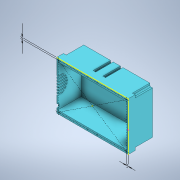
# Autodesk Inventor part: caseUpperPortion
Saved by Autodesk Inventor 2022.1 (Build 261234020, 234B)
## iProperties
Created: 2021-08-20
Part Number: caseUpperPortion
Material: PC/ABS Plastic
Document SubType Name: Modeling
Designer: robst
Density: 0.357273 g/cm^3
Appearance: Cadet Blue
Author: robst
Autodesk Inventor part; units mm, degrees
ref_plane "YZ Plane" through (0, 0, 0) normal (1, 0, 0) x (0, 1, 0)
ref_plane "XZ Plane" through (0, 0, 0) normal (0, 1, 0) x (-1, 0, 0)
ref_plane "XY Plane" through (0, 0, 0) normal (0, 0, 1) x (1, 0, 0)
sketch "Sketch1" plane through (0, 0, 0) normal (0, 0, 1) x (1, 0, 0)
  line L0 (-110.35, -74.5) -> (110.35, -74.5)
  line L1 (110.35, -74.5) -> (110.35, 74.5)
  line L2 (110.35, 74.5) -> (-110.35, 74.5)
  line L3 (-110.35, 74.5) -> (-110.35, -74.5)
  line L4 (-110.35, -74.5) -> (110.35, 74.5) construction
  line L5 (110.35, -74.5) -> (-110.35, 74.5) construction
  point P0 (0, 0)
  dimension "d0" = 220.7
  dimension "d1" = 149
  constraints: 12 end point, 2 midpoint, 2 parallel, 1 horizontal, 1 perpendicular
  measures "d0" distance of L0.start L0.end
  measures "d1" distance of L1.end L0.end
extrude "MainInnerBodyExtrusion" add sketch "Sketch1" against normal blind 75
sketch "Sketch3" plane through (0, 0, 0) normal (0, 0, 1) x (1, 0, 0)
  line L0 (37.65, -26) -> (94.65, -26)
  line L1 (94.65, -26) -> (94.65, 26)
  line L2 (94.65, 26) -> (37.65, 26)
  line L3 (37.65, 26) -> (37.65, -26)
  line L4 (37.65, -26) -> (94.65, 26) construction
  line L5 (94.65, -26) -> (37.65, 26) construction
  line L6 (110.35, -74.5) -> (110.35, 74.5) projected
  line L7 (0, 0) -> (110.35, 0) construction
  line L8 (-110.35, -74.5) -> (-110.35, 74.5) construction
  line L9 (-110.35, 74.5) -> (-110.35, -74.5) projected
  point P0 (66.15, 0)
  point P1 (66.15, 0)
  dimension "d5" = 15.7
  dimension "d6" = 52
  dimension "d7" = 57
  constraints: 14 end point, 4 midpoint, 2 parallel, 1 horizontal, 1 perpendicular, 1 point on line
  measures "d5" distance between parallel lines of L1 L6
  measures "d6" distance of L0.end L1.end
  measures "d7" distance of L1.end L2.end
extrude "HoleForCamerabase" cut sketch "Sketch3" against normal blind 47
sketch "Sketch4" plane through (0, 0, 0) normal (0, 0, 1) x (1, 0, 0)
  line L0 (0, 0) -> (-110.35, 0) construction
  line L1 (-110.35, -74.5) -> (-110.35, 74.5) construction
  line L2 (-107.35, -31) -> (-91.35, -31)
  line L3 (-91.35, -31) -> (-91.35, 31)
  line L4 (-91.35, 31) -> (-107.35, 31)
  line L5 (-107.35, 31) -> (-107.35, -31)
  line L6 (-107.35, -31) -> (-91.35, 31) construction
  line L7 (-91.35, -31) -> (-107.35, 31) construction
  point P0 (-99.35, 0)
  dimension "d13" = 16
  dimension "d14" = 62
  dimension "d15" = 3
  constraints: 14 end point, 3 midpoint, 2 parallel, 1 perpendicular, 1 point on line
  measures "d13" distance of L2.start L2.end
  measures "d14" distance of L3.end L2.end
  measures "d15" distance between parallel lines of L1 L5
extrude "HoleForFan" cut sketch "Sketch4" against normal blind 47
sketch "Sketch15" plane through (-110.35, -74.5, 0) normal (-1, 0, 0) x (0, 0, 1)
  line L0 (0, 149) -> (0, 0) projected
  line L1 (0, 149) -> (-75, 149) projected
  line L2 (-75, 0) -> (-75, 149) projected
  line L3 (0, 0) -> (-75, 0) projected
  line L4 (0, 0) -> (0, 149) projected
  line L5 (0, 100.5) -> (0, 48.5) projected
  line L6 (0, 74.5) -> (-30, 74.5) construction
  line L7 (0, 76.5) -> (-29.9333, 76.5)
  line L8 (0, 84.5) -> (-28.2843, 84.5)
  line L9 (0, 80.5) -> (-29.3939, 80.5)
  line L10 (0, 76.5) -> (0, 74.5)
  line L11 (0, 88.5) -> (-26.533, 88.5)
  line L12 (0, 92.5) -> (-24, 92.5)
  line L13 (-20.3961, 96.5) -> (0, 96.5)
  line L14 (-14.9666, 100.5) -> (0, 100.5)
  line L15 (0, 84.5) -> (0, 80.5)
  line L16 (0, 100.5) -> (0, 96.5)
  line L17 (0, 92.5) -> (0, 88.5)
  line L18 (0, 72.5) -> (-29.9333, 72.5)
  line L19 (0, 64.5) -> (-28.2843, 64.5)
  line L20 (0, 68.5) -> (-29.3939, 68.5)
  line L21 (0, 72.5) -> (0, 74.5)
  line L22 (0, 60.5) -> (-26.533, 60.5)
  line L23 (0, 56.5) -> (-24, 56.5)
  line L24 (-20.3961, 52.5) -> (0, 52.5)
  line L25 (-14.9666, 48.5) -> (0, 48.5)
  line L26 (0, 64.5) -> (0, 68.5)
  line L27 (0, 56.5) -> (0, 60.5)
  line L28 (0, 48.5) -> (0, 52.5)
  line L29 (0, 72.5) -> (0, 76.5)
  line L30 (0, 80.5) -> (0, 84.5)
  line L31 (0, 88.5) -> (0, 92.5)
  line L32 (0, 96.5) -> (0, 149)
  arc A0 (-28.2843, 84.5) -> (-29.3939, 80.5) centre (0, 74.5) ccw
  arc A1 (-14.9666, 100.5) -> (-20.3961, 96.5) centre (0, 74.5) ccw
  arc A2 (-24, 92.5) -> (-26.533, 88.5) centre (0, 74.5) ccw
  arc A3 (-29.9333, 76.5) -> (-29.9333, 72.5) centre (0, 74.5) ccw
  arc A4 (-29.3939, 68.5) -> (-28.2843, 64.5) centre (0, 74.5) ccw
  arc A5 (-26.533, 60.5) -> (-24, 56.5) centre (0, 74.5) ccw
  arc A6 (-20.3961, 52.5) -> (-14.9666, 48.5) centre (0, 74.5) ccw
  point P0 (0, 74.5)
  point P1 (0, 82)
  point P2 (0, 67.0167)
  point P3 (0, 4.25)
  point P4 (-10.198, 96.5)
  point P5 (0, 48.5)
  point P6 (0, 52.5)
  point P7 (0, 56.5)
  point P8 (0, 60.5)
  point P9 (0, 64.5)
  point P10 (0, 68.5)
  point P11 (0, 72.5)
  point P12 (0, 80.5)
  point P13 (0, 84.5)
  point P14 (0, 88.5)
  point P15 (0, 92.5)
  point P16 (0, 96.5)
  point P17 (0, 100.5)
  dimension "d69" = 2
  dimension "d71" = 4
  dimension "d72" = 4
  dimension "d73" = 4
  dimension "d75" = 4
  dimension "d142" = 30
  constraints: 54 end point, 15 point on circle, 15 symmetric about line, 7 centre point, 3 parallel, 3 perpendicular, 2 horizontal, 1 coincident, 1 midpoint, 1 other
  measures "d69" distance between parallel lines of L7 L6
  measures "d71" distance between parallel lines of L8 L9
  measures "d72" distance between parallel lines of L11 L8
  measures "d73" distance between parallel lines of L12 L11
  measures "d75" distance between parallel lines of L13 L14
  measures "d142" radius of A2
extrude "SlotsForRearFan" cut sketch "Sketch15" against normal up to surface (3 mm away) contours L0 L13 A1 L14 | L0 L11 A2 L12 | L25 A6 L24 L0 | L0 L9 A0 L8 | L23 A5 L22 L0 | L0 L18 A3 L7 | L19 A4 L20 L0
sketch "Sketch16" plane through (0, 0, -47) normal (0, 0, 1) x (1, 0, 0)
  line L0 (94.65, 26) -> (94.65, -26) projected
  line L1 (79.15, 10.765) -> (79.15, -11.235) construction
  line L2 (77.65, 10.765) -> (77.65, -11.235)
  line L3 (74.65, -11.235) -> (74.65, 10.765)
  line L4 (71.65, 8.7746) -> (71.65, -9.2446)
  line L5 (68.65, 3.5785) -> (68.65, -4.0485)
  line L6 (80.65, 10.765) -> (80.65, -11.235)
  line L7 (83.65, -11.235) -> (83.65, 10.765)
  line L8 (86.65, 8.7746) -> (86.65, -9.2446)
  line L9 (89.65, 3.5785) -> (89.65, -4.0485)
  line L10 (72.7991, 10.765) -> (74.65, 10.765)
  line L11 (74.65, -11.235) -> (72.7991, -11.235)
  line L12 (72.7991, -11.235) -> (71.65, -9.2446)
  line L13 (68.65, -4.0485) -> (66.4483, -0.235)
  line L14 (66.4483, -0.235) -> (68.65, 3.5785)
  line L15 (71.65, 8.7746) -> (72.7991, 10.765)
  line L16 (77.65, 10.765) -> (80.65, 10.765)
  line L17 (83.65, 10.765) -> (85.5009, 10.765)
  line L18 (85.5009, -11.235) -> (83.65, -11.235)
  line L19 (80.65, -11.235) -> (77.65, -11.235)
  line L20 (91.8517, -0.235) -> (89.65, -4.0485)
  line L21 (86.65, -9.2446) -> (85.5009, -11.235)
  line L22 (85.5009, 10.765) -> (86.65, 8.7746)
  line L23 (89.65, 3.5785) -> (91.8517, -0.235)
  point P0 (0, 0)
  point P1 (79.15, -0.235)
  point P2 (68.65, -0.235)
  dimension "d78" = 15.5
  dimension "d89" = 1.5
  dimension "d90" = 3
  dimension "d91" = 3
  dimension "d92" = 3
  constraints: 46 end point, 8 symmetric about line, 6 perpendicular, 3 horizontal, 3 midpoint, 2 vertical, 7 other
  measures "d78" distance from line of point (79.15, -0.235) L0
  measures "d89" distance between parallel lines of L2 L1
  measures "d90" distance between parallel lines of L3 L2
  measures "d91" distance between parallel lines of L4 L3
  measures "d92" distance from line of point (68.65, -0.235) L4
extrude "VentForCamera" cut sketch "Sketch16" against normal through all
sketch "Sketch23" plane through (0, 0, 0) normal (0, 0, 1) x (1, 0, 0)
  line L0 (-105.35, -69.5) -> (105.35, -69.5) construction
  line L1 (105.35, -69.5) -> (105.35, 69.5) construction
  line L2 (105.35, 69.5) -> (-105.35, 69.5) construction
  line L3 (-105.35, 69.5) -> (-105.35, -69.5) construction
  line L4 (-105.35, -69.5) -> (105.35, 69.5) construction
  line L5 (105.35, -69.5) -> (-105.35, 69.5) construction
  line L6 (110.35, -74.5) -> (110.35, 74.5) projected
  line L7 (110.35, 74.5) -> (-110.35, 74.5) projected
  point P0 (0, 0)
  point P1 (110.35, -8)
  dimension "d106" = 5
  dimension "d108" = 5
  constraints: 12 end point, 4 coincident, 2 midpoint, 2 parallel, 1 horizontal, 1 perpendicular
  measures "d106" distance between parallel lines of L1 L6
  measures "d108" distance between parallel lines of L2 L7
hole "Screw hole for 6-32 screw" at (-105.35, -69.5, 0) at (105.35, -69.5, 0) at (105.35, 69.5, 0) at (-105.35, 69.5, 0) direction (0, 0, -1) diameter 4.051 end through all clearance for "Hex Machine Screw" size "#6" standard "Ansi Unified Screw Threads"
sketch "Sketch26" plane through (-110.35, -74.5, -75) normal (-1, 0, 0) x (0, 0, 1)
  line L0 (75, 139) -> (75, 111) projected
  circle A0 centre (75, 20) radius 6
  line L1 (75, 0) -> (0, 0) projected
  point P0 (75, 74.5)
  point P1 (50, 139)
  point P2 (50, 10)
  dimension "d143" = 20
  dimension "d144" = 12
  constraints: 1 centre point, 2 other
  measures "d143" distance from line of A0.centre L1
  measures "d144" diameter of A0
extrude "Extrusion19" cut sketch "Sketch26" against normal up to surface (3 mm away)
sketch "Sketch28" plane through (0, 0, -75) normal (0, 0, -1) x (-1, 0, 0)
  circle A0 centre (-105.35, -69.5) radius 2.0255 projected
  circle A1 centre (-105.35, 69.5) radius 2.0255 projected
  circle A2 centre (105.35, 69.5) radius 2.0255 projected
  circle A3 centre (105.35, -69.5) radius 2.0255 projected
  circle A4 centre (-105.35, -69.5) radius 2.0255 projected
  circle A5 centre (-105.35, -69.5) radius 3.5
  circle A6 centre (-105.35, 69.5) radius 3.5
  circle A7 centre (105.35, 69.5) radius 3.5
  circle A8 centre (105.35, -69.5) radius 3.5
  point P0 (0, 0)
  dimension "d150" = 7
  constraints: 4 centre point, 4 coincident, 3 equal radius
  measures "d150" diameter of A5
extrude "Extrusion21" cut sketch "Sketch28" against normal blind 58 contours A1 | A2 | A3 | A5 | A6 | A7 | A8
sketch "Sketch29" plane through (0, 0, 0) normal (0, 0, 1) x (1, 0, 0)
  line L0 (107.35, -64.5) -> (107.35, 64.5)
  line L1 (107.35, 64.5) -> (-107.35, 64.5)
  line L2 (-107.35, 64.5) -> (-107.35, -64.5)
  line L3 (-107.35, -64.5) -> (107.35, -64.5)
  line L4 (107.35, -64.5) -> (-107.35, 64.5) construction
  line L5 (107.35, 64.5) -> (-107.35, -64.5) construction
  line L6 (-110.35, -74.5) -> (110.35, -74.5) projected
  line L7 (-110.35, 74.5) -> (-110.35, 26) projected
  point P0 (0, 0)
  dimension "d153" = 10
  dimension "d154" = 3
  constraints: 12 end point, 2 midpoint, 2 parallel, 1 perpendicular, 1 vertical
  measures "d153" distance between parallel lines of L6 L3
  measures "d154" distance between parallel lines of L2 L7
extrude "Extrusion22" cut sketch "Sketch29" against normal blind 72
sketch "Sketch30" plane through (0, 0, -75) normal (0, 0, -1) x (-1, 0, 0)
  circle A0 centre (-105.35, -69.5) radius 2.0255 construction
  line L0 (-105.35, -69.5) -> (107.35, -69.5) construction
  circle A1 centre (-105.35, 69.5) radius 2.0255 construction
  line L1 (-105.35, 69.5) -> (105.3316, 69.5) construction
  line L2 (107.35, 64.5) -> (-107.35, 64.5) construction
  line L3 (15, -69.5) -> (15, 69.5) construction
  line L4 (15, 69.5) -> (-15, 69.5) construction
  line L5 (-15, 69.5) -> (-15, -69.5) construction
  line L6 (-15, -69.5) -> (15, -69.5) construction
  line L7 (15, -69.5) -> (-15, 69.5) construction
  line L8 (15, 69.5) -> (-15, -69.5) construction
  point P0 (0, 0)
  dimension "d157" = 30
  constraints: 16 end point, 4 coincident, 3 parallel, 2 midpoint, 1 horizontal, 1 perpendicular, 1 vertical
  measures "d157" distance of L4.end L3.end
hole "Hole5" at (15, -69.5, -75) at (15, 69.5, -75) at (-15, 69.5, -75) at (-15, -69.5, -75) direction (0, 0, 1) diameter 4.051 end through all counterbore diameter 8 counterbore depth 58 clearance for "Hex Machine Screw" size "#6" standard "Ansi Unified Screw Threads"
sketch "Sketch31" plane through (0, 0, -75) normal (0, 0, -1) x (-1, 0, 0)
  circle A0 centre (105.35, 69.5) radius 2.0255 construction
  circle A1 centre (15, -69.5) radius 2.0255 construction
  line L0 (105.35, 69.5) -> (15, 69.5) construction
  line L1 (15, 69.5) -> (15, -69.5) construction
  line L2 (15, -69.5) -> (105.35, -69.5) construction
  line L3 (105.35, -69.5) -> (105.35, 69.5) construction
  circle A2 centre (-15, 69.5) radius 2.0255 construction
  circle A3 centre (-105.35, -69.5) radius 2.0255 construction
  line L4 (-15, 69.5) -> (-105.35, 69.5) construction
  line L5 (-105.35, 69.5) -> (-105.35, -69.5) construction
  line L6 (-105.35, -69.5) -> (-15, -69.5) construction
  line L7 (-15, -69.5) -> (-15, 69.5) construction
  circle A4 centre (-105.35, 69.5) radius 2.0255 projected
  line L8 (-110.35, 74.5) -> (-100.35, 64.5) construction
  line L9 (-110.35, 64.5) -> (-100.35, 74.5) construction
  line L10 (110.35, 74.5) -> (-110.35, 74.5) projected
  line L11 (-110.35, 74.5) -> (-110.35, -74.5) projected
  line L12 (-110.35, 74.5) -> (-110.35, 66)
  line L13 (-110.35, 66) -> (-101.85, 66)
  line L14 (-101.85, 66) -> (-101.85, 74.5)
  line L15 (-101.85, 74.5) -> (-110.35, 74.5)
  circle A5 centre (-105.35, 69.5) radius 3.5 projected
  circle A6 centre (-15, 69.5) radius 4 projected
  line L16 (-11, 69.5) -> (-11, 74.5)
  line L17 (-11, 74.5) -> (-19, 74.5)
  line L18 (-19, 69.5) -> (-19, 74.5)
  point P0 (0, 0)
  point P1 (-105.35, 66)
  point P2 (-101.85, 69.5)
  constraints: 34 end point, 6 perpendicular, 4 parallel, 4 tangent, 3 collinear, 3 horizontal, 2 midpoint, 2 point on circle, 2 point on line, 1 vertical
extrude "Extrusion24" cut sketch "Sketch31" against normal blind 54 contours L14 A5 L13 L11 L10
mirror "Mirror2" about plane through (0, 0, 0) normal (0, 1, 0) of "Extrusion24"
mirror "Mirror3" about plane through (0, 0, 0) normal (1, 0, 0) of "Extrusion24", "Mirror2"
extrude "Extrusion25" cut sketch "Sketch31" against normal blind 54 contours L16 A6 L18 L10
mirror "Mirror4" about plane through (0, 0, 0) normal (0, 1, 0) of "Extrusion25"
mirror "Mirror5" about plane through (0, 0, 0) normal (1, 0, 0) of "Extrusion25", "Mirror4"
sketch "Sketch32" plane through (0, 0, -72) normal (0, 0, 1) x (1, 0, 0)
  point P0 (27.81, 58)
  point P1 (27.81, -58)
hole "Hole6" at (27.81, 58, -72) at (27.81, -58, -72) direction (0, 0, -1) diameter 5.1054 depth 3
equation "\"d0\" = newCaseLength"
equation "\"d1\" = caseWidth"
equation "\"d5\" = lensLength"
equation "\"d6\" = cameraWidth"
equation "\"d7\" = cameraLength"
equation "\"d8\" = maxComponentDepth"
equation "\"d13\" = fanDepth"
equation "\"d14\" = fanWidth"
equation "\"d15\" = rearWallThickness"
equation "\"d16\" = maxComponentDepth"
equation "\"caseWidth\" = piCaseLength + 2 * outsideWallThickness"
equation "\"oneHalfCaseDepth\" = piCaseWidth"
equation "\"cameraDepth\" = 61"
equation "\"caseLength\" = 189.7"
equation "\"lensLength\" = 15.7"
equation "\"piCaseWidth\" = 63"
equation "\"piCaseDepth\" = 32"
equation "\"poeDepth\" = 38"
equation "\"piEthernetCableReliefLength\" = 35"
equation "\"poeEthernetCableReliefLength\" = 35"
equation "\"thermisterDepth\" = 18"
equation "\"sensorDepth\" = 11"
equation "\"cutoutDepth\" = 0.5 * piCaseWidth"
equation "\"thickenDistance\" = 1"
equation "\"bottomOfCaseWallThickness\" = 3"
equation "\"rearWallThickness\" = 3"
equation "\"maxComponentDepth\" = extraCutoutDepth + 0.5 * piCaseWidth"
equation "\"caseDepth\" = 75"
equation "\"minDelta\" = 16"
equation "\"fanCutoutDepth\" = 0.5 * fanLength + extraCutoutDepth + thickenDistance"
equation "\"newCaseLength\" = cameraLength + piCaseDepth + fanDepth + poeWidth + rearWallThickness + 3 * minDelta + lensLength"
equation "\"frontWallThickness\" = 3"
equation "\"d95\" = lensDiameter"
equation "\"extraCutoutDepth\" = 15.5"
equation "\"cameraWidth\" = 52"
equation "\"cameraLength\" = 57"
equation "\"fanDepth\" = 16"
equation "\"fanWidth\" = 62"
equation "\"piCaseLength\" = 129"
equation "\"outsideWallThickness\" = 10"
equation "\"fanLength\" = 60"
equation "\"poeWidth\" = 49"
equation "\"lensDiameter\" = 15"
body "Solid1"
